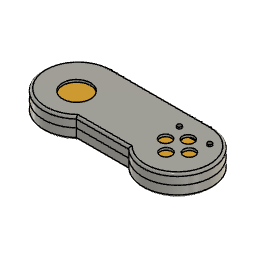
Controller v45 (Autodesk Fusion 360 design; units mm, degrees)
Autodesk Fusion 360 part; units mm, degrees
(part 1 of 2)
sketch "Skizze1" plane through (0, 0, 0) normal (0, 0, 1) x (1, 0, 0)
  line L0 (-75, 23.3) -> (75, 23.3)
  line L1 (75, 23.3) -> (75, -23.3)
  line L2 (75, -23.3) -> (-75, -23.3)
  line L3 (-75, -23.3) -> (-75, 23.3)
  line L4 (-71.7, -23.3) -> (-71.7, -14) construction
  line L5 (-75, -20) -> (-63, -20) construction
  circle A0 centre (-70.1, -18.4) radius 1.6
  line L6 (0, 1.75) -> (0, 22.5) construction
  circle A1 centre (70.1, -18.4) radius 1.6
  line L7 (0, 23.3) -> (0, 21.05) construction
  line L8 (0, 21.05) -> (0, 19.45) construction
  circle A2 centre (0, 19.45) radius 1.6
  line L9 (66.75, 19.8) -> (72.65, 19.8) construction
  line L10 (72.65, 19.8) -> (72.65, 13.9) construction
  line L11 (72.65, 13.9) -> (66.75, 13.9) construction
  line L12 (66.75, 13.9) -> (66.75, 19.8) construction
  line L13 (69.7, 19.8) -> (69.7, 13.9) construction
  circle A3 centre (69.7, 16.85) radius 2.5
  line L14 (34.15, 19.8) -> (40.05, 19.8) construction
  line L15 (40.05, 19.8) -> (40.05, 13.9) construction
  line L16 (40.05, 13.9) -> (34.15, 13.9) construction
  line L17 (34.15, 13.9) -> (34.15, 19.8) construction
  line L18 (37.1, 19.8) -> (37.1, 13.9) construction
  circle A4 centre (37.1, 16.85) radius 2.5
  line L19 (47.25, 16.2) -> (59.15, 16.2) construction
  line L20 (59.15, 16.2) -> (59.15, 4.3) construction
  line L21 (59.15, 4.3) -> (47.25, 4.3) construction
  line L22 (47.25, 4.3) -> (47.25, 16.2) construction
  line L23 (47.25, -7.6) -> (59.15, -7.6) construction
  line L24 (59.15, -7.6) -> (59.15, -19.5) construction
  line L25 (59.15, -19.5) -> (47.25, -19.5) construction
  line L26 (47.25, -19.5) -> (47.25, -7.6) construction
  line L27 (60.1, 4.6) -> (72, 4.6) construction
  line L28 (72, 4.6) -> (72, -7.3) construction
  line L29 (72, -7.3) -> (60.1, -7.3) construction
  line L30 (60.1, -7.3) -> (60.1, 4.6) construction
  line L31 (34.5, 4.6) -> (46.4, 4.6) construction
  line L32 (46.4, 4.6) -> (46.4, -7.3) construction
  line L33 (46.4, -7.3) -> (34.5, -7.3) construction
  line L34 (34.5, -7.3) -> (34.5, 4.6) construction
  line L35 (53.2, 16.2) -> (53.2, 4.3) construction
  line L36 (40.45, 4.6) -> (40.45, -7.3) construction
  line L37 (66.05, 4.6) -> (66.05, -7.3) construction
  line L38 (53.2, -7.6) -> (53.2, -19.5) construction
  circle A5 centre (40.45, -1.35) radius 6.25
  circle A6 centre (53.2, 10.25) radius 6.25
  circle A7 centre (66.05, -1.35) radius 6.25
  circle A8 centre (53.2, -13.55) radius 6.25
  line L39 (-59.6, 3.4) -> (-43.6, 3.4) construction
  line L40 (-43.6, 3.4) -> (-43.6, -12.6) construction
  line L41 (-43.6, -12.6) -> (-59.6, -12.6) construction
  line L42 (-59.6, -12.6) -> (-59.6, 3.4) construction
  line L43 (-51.6, 3.4) -> (-51.6, -12.6) construction
  circle A9 centre (-51.6, -4.6) radius 15
  dimension "d9" = 75
  dimension "d10" = 23.3
  dimension "d11" = 150
  dimension "d12" = 46.6
  dimension "d14" = 3.3
  dimension "d15" = 3.3
  dimension "d16" = 3.2
  dimension "d17" = 2.25
  dimension "d19" = 1.6
  dimension "d20" = 3.2
  dimension "d21" = 5.9
  dimension "d22" = 5.9
  dimension "d23" = 3.5
  dimension "d24" = 2.35
  dimension "d25" = 5
  dimension "d26" = 5.9
  dimension "d27" = 5.9
  dimension "d28" = 3.5
  dimension "d29" = 26.7
  dimension "d30" = 5
  dimension "d33" = 11.9
  dimension "d34" = 11.9
  dimension "d35" = 7.6
  dimension "d36" = 7.1
  dimension "d37" = 11.9
  dimension "d38" = 11.9
  dimension "d39" = 11.9
  dimension "d40" = 11.9
  dimension "d41" = 11.9
  dimension "d42" = 11.9
  dimension "d43" = 11.9
  dimension "d44" = 3
  dimension "d45" = 13.7
  dimension "d46" = 9.3
  dimension "d47" = 12.5
  dimension "d48" = 12.5
  dimension "d49" = 12.5
  dimension "d50" = 12.5
  dimension "d51" = 16
  dimension "d52" = 16
  dimension "d53" = 15.4
  dimension "d54" = 10.7
  dimension "d56" = 30
  constraint horizontal L0
  constraint vertical L1
  constraint horizontal L2
  constraint vertical L3
  constraint coincident L2 L4.start
  constraint perpendicular L2 L4
  constraint coincident L3 L5.start
  constraint perpendicular L3 L5
  constraint tangent L5 A0
  constraint tangent L4 A0
  constraint symmetric A0 L6 A1
  constraint midpoint L0 L7.start
  constraint perpendicular L0 L7
  constraint parallel L6 L8
  constraint coincident L8.end A2.centre
  constraint horizontal L9
  constraint vertical L10
  constraint horizontal L11
  constraint vertical L12
  constraint midpoint L9 L13.start
  constraint midpoint L11 L13.end
  constraint midpoint L13 A3.centre
  constraint horizontal L14
  constraint vertical L15
  constraint horizontal L16
  constraint vertical L17
  constraint midpoint L14 L18.start
  constraint midpoint L16 L18.end
  constraint midpoint L18 A4.centre
  constraint horizontal L19
  constraint vertical L20
  constraint horizontal L21
  constraint vertical L22
  constraint horizontal L23
  constraint vertical L24
  constraint horizontal L25
  constraint vertical L26
  constraint horizontal L27
  constraint vertical L28
  constraint horizontal L29
  constraint vertical L30
  constraint horizontal L31
  constraint vertical L32
  constraint horizontal L33
  constraint vertical L34
  constraint collinear L22 L26
  constraint collinear L27 L31
  constraint midpoint L19 L35.start
  constraint midpoint L21 L35.end
  constraint midpoint L31 L36.start
  constraint midpoint L33 L36.end
  constraint midpoint L27 L37.start
  constraint midpoint L29 L37.end
  constraint midpoint L23 L38.start
  constraint midpoint L25 L38.end
  constraint midpoint L36 A5.centre
  constraint midpoint L35 A6.centre
  constraint midpoint L37 A7.centre
  constraint midpoint L38 A8.centre
  constraint horizontal L39
  constraint vertical L40
  constraint horizontal L41
  constraint vertical L42
  constraint midpoint L39 L43.start
  constraint midpoint L41 L43.end
  constraint midpoint L43 A9.centre
  measures "d9" distance of origin L3
  measures "d10" distance of origin L0
  measures "d11" distance of L0.start L0.end
  measures "d12" distance of L0.start L2.end
  measures "d14" distance of L3 L4
  measures "d15" distance of L2 L5
  measures "d16" diameter of A0
  measures "d17" distance of L7.start L7.end
  measures "d19" distance of L7.end L8.end
  measures "d20" diameter of A2
  measures "d21" distance of L9.start L9.end
  measures "d22" distance of L9.start L11.end
  measures "d23" distance of L0 L9
  measures "d24" distance of L1 L10
  measures "d25" diameter of A3
  measures "d26" distance of L14.start L14.end
  measures "d27" distance of L14.start L16.end
  measures "d28" distance of L0 L14
  measures "d29" distance of L12 L15
  measures "d30" diameter of A4
  measures "d33" distance of L19.start L19.end
  measures "d34" distance of L19.start L21.end
  measures "d35" distance of L12 L20
  measures "d36" distance of L0 L19
  measures "d37" distance of L23.start L23.end
  measures "d38" distance of L23.start L25.end
  measures "d39" distance of L27.start L27.end
  measures "d40" distance of L27.start L29.end
  measures "d41" distance of L31.start L31.end
  measures "d42" distance of L31.start L33.end
  measures "d43" distance of L21 L23
  measures "d44" distance of L1 L28
  measures "d45" distance of L30 L32
  measures "d46" distance of L11 L27
  measures "d47" diameter of A5
  measures "d48" diameter of A6
  measures "d49" diameter of A7
  measures "d50" diameter of A8
  measures "d51" distance of L39.start L39.end
  measures "d52" distance of L39.start L41.end
  measures "d53" distance of L3 L42
  measures "d54" distance of L2 L41
  measures "d56" diameter of A9
sketch "Skizze2" plane through (0, 0, 0) normal (0, 0, 1) x (1, 0, 0)
  circle A0 centre (-51.6, -4.6) radius 15
  circle A1 centre (40.45, -1.35) radius 6.25
  circle A2 centre (53.2, 10.25) radius 6.25
  circle A3 centre (66.05, -1.35) radius 6.25
  circle A4 centre (53.2, -13.55) radius 6.25
  circle A5 centre (69.7, 16.85) radius 2.5
  circle A6 centre (37.1, 16.85) radius 2.5
  circle A7 centre (70.1, -18.4) radius 1.6
  circle A8 centre (0, 19.45) radius 1.6
  circle A9 centre (-70.1, -18.4) radius 1.6
  line L0 (-75, -23.3) -> (-75, 23.3)
  line L1 (-75, 23.3) -> (75, 23.3)
  line L2 (75, 23.3) -> (75, -23.3)
  line L3 (75, -23.3) -> (-75, -23.3)
  line L4 (40.45, -1.35) -> (66.05, -1.35) construction
  line L5 (53.2, 10.25) -> (53.2, -13.55) construction
  circle A10 centre (53.25, -1.35) radius 32.8738 construction
  line L6 (0, 87.6668) -> (0, -41.0668) construction
  circle A11 centre (53.25, -1.35) radius 36.8738 construction
  line L7 (53.25, 35.5238) -> (0, 35.5238)
  line L8 (28.0831, -28.3) -> (0, -28.3)
  arc A12 (28.0831, -28.3) -> (53.25, 35.5238) centre (53.25, -1.35) ccw
  line L9 (-53.25, 35.5238) -> (0, 35.5238)
  arc A13 (-53.25, 35.5238) -> (-28.0831, -28.3) centre (-53.25, -1.35) ccw
  line L10 (-28.0831, -28.3) -> (0, -28.3)
  dimension "d59" = 4
  dimension "d60" = 5
  constraint coincident A1.centre L4.start
  constraint coincident A3.centre L4.end
  constraint coincident A2.centre L5.start
  constraint coincident A4.centre L5.end
  constraint midpoint L4 A10.centre
  constraint coincident L1.end A10
  constraint perpendicular L3 L6
  constraint midpoint L1 L6
  constraint coincident A11 L7.start
  constraint coincident L6 L7.end
  constraint tangent A11 L7
  constraint coincident A11 L8.start
  constraint coincident L6 L8.end
  constraint perpendicular L6 L8
  constraint perpendicular L6 L7
  constraint tangent L7 A12
  constraint symmetric L6 L7.start L9.start
  constraint symmetric L6 L7.end L9.end
  constraint symmetric L6 L8.start A13.end
  constraint symmetric L6 L8.end L10.end
  constraint symmetric L6 A12 A13
  measures "d60" distance of L3 L8
sketch "Skizze3" plane through (0, 0, 0) normal (0, 0, 1) x (1, 0, 0)
  line L0 (-53.25, 35.5238) -> (0, 35.5238)
  arc A0 (-53.25, 35.5238) -> (-28.0831, -28.3) centre (-53.25, -1.35) ccw
  line L1 (-28.0831, -28.3) -> (0, -28.3)
  line L2 (28.0831, -28.3) -> (0, -28.3)
  arc A1 (28.0831, -28.3) -> (53.25, 35.5238) centre (53.25, -1.35) ccw
  line L3 (53.25, 35.5238) -> (0, 35.5238)
  line L4 (-75, 23.3) -> (75, 23.3) construction
  line L5 (-75, -23.3) -> (-75, 23.3) construction
  line L6 (75, -23.3) -> (-75, -23.3) construction
  line L7 (75, 23.3) -> (75, -23.3) construction
  arc A2 (-53.25, 33.0238) -> (-29.089, -25.8) centre (-53.25, -1.35) ccw
  line L8 (-29.089, -25.8) -> (0, -25.8)
  line L9 (29.089, -25.8) -> (0, -25.8)
  arc A3 (29.089, -25.8) -> (53.25, 33.0238) centre (53.25, -1.35) ccw
  line L10 (53.25, 33.0238) -> (0, 33.0238)
  line L11 (-53.25, 33.0238) -> (0, 33.0238)
  circle A4 centre (-70.1, -18.4) radius 1.25
  circle A5 centre (-70.1, -18.4) radius 3
  circle A6 centre (0, 19.45) radius 1.5
  circle A7 centre (0, 19.45) radius 3
  circle A8 centre (70.1, -18.4) radius 3
  circle A9 centre (70.1, -18.4) radius 1.25
  circle A10 centre (0, 19.45) radius 5.5
  circle A11 centre (-70.1, -18.4) radius 5.5
  circle A12 centre (70.1, -18.4) radius 5.5
  circle A13 centre (83.25, 0) radius 2.75
  circle A14 centre (83.25, 0) radius 1.75
  line L12 (78, 22.5036) -> (78, -25.2036)
  line L13 (0, -28.3) -> (0, 35.5238) construction
  line L14 (-78, 22.5036) -> (-78, -25.2036)
  circle A15 centre (-83.25, 0) radius 2.75
  circle A16 centre (-83.25, 0) radius 1.75
  point P0 (0, 19.45)
  point P1 (70.1, -18.4)
  point P2 (-70.1, -18.4)
  dimension "d62" = 2.5
  dimension "d63" = 6
  dimension "d64" = 3
  dimension "d65" = 6
  dimension "d66" = 6
  dimension "d67" = 2.5
  dimension "d69" = 2.5
  dimension "d70" = 2.5
  dimension "d71" = 2.5
  dimension "d257" = 5.5
  dimension "d258" = 3.5
  dimension "d261" = 3
  dimension "d262" = 5.25
  constraint coincident P2 A4.centre
  constraint coincident P0 A6.centre
  constraint concentric A6 A7
  constraint coincident P1 A8.centre
  constraint concentric A8 A9
  constraint concentric A13 A14
  constraint coincident A3 L12.start
  constraint coincident A3 L12.end
  constraint vertical L12
  constraint coincident L1.end L2.end
  constraint coincident L0.end L3.end
  constraint symmetric A13 L13 A15
  constraint symmetric A14 L13 A16
  constraint symmetric L12.start L13 L14.start
  constraint symmetric L12.end L13 L14.end
  measures "d62" diameter of A4
  measures "d63" diameter of A5
  measures "d64" diameter of A6
  measures "d65" diameter of A7
  measures "d66" diameter of A8
  measures "d67" diameter of A9
  measures "d257" diameter of A13
  measures "d258" diameter of A14
  measures "d261" distance of L7 L12
  measures "d262" distance of A13.centre L12
extrude "Extrusion1" add sketch "Skizze3" along normal blind 2.5 contours A2 L8 L9 A3 L10 L11 L12 L14 | A2 L14 | A3 L12 makes body 1
extrude "Extrusion2" add sketch "Skizze3" along normal blind 10 contours A5 | A7 | A8 | A10 | A11 | A12 bodies 1
extrude "Extrusion3" cut sketch "Skizze3" along normal blind 6.25 contours A5 | A7 | A8 bodies 1
extrude "Extrusion4" add sketch "Skizze3" along normal blind 11.5 separate body contours L0 A0 L1 L2 A1 L3 | A2 L14 | A3 L12 | A13 | A14 | A15 | A16 makes body 2
extrude "Extrusion28" cut sketch "Skizze3" along normal blind 11.5 contours A14 | A16 bodies 2
extrude "Extrusion29" cut sketch "Skizze3" along normal blind 5 contours A13 | A15 bodies 2
sketch "Skizze4" plane through (0, 0, 10) normal (0, 0, 1) x (-1, 0, 0)
  circle A0 centre (0, -19.45) radius 1.5
  circle A1 centre (0, -19.45) radius 5.5
  line L0 (75, -23.3) -> (-75, -23.3)
  line L1 (75, 23.3) -> (75, -23.3)
  line L2 (-75, 23.3) -> (75, 23.3)
  line L3 (-75, -23.3) -> (-75, 23.3)
  circle A2 centre (-37.1, -16.85) radius 2.5
  circle A3 centre (-53.2, -10.25) radius 6.25
  circle A4 centre (-69.7, -16.85) radius 2.5
  circle A5 centre (-66.05, 1.35) radius 6.25
  circle A6 centre (-40.45, 1.35) radius 6.25
  circle A7 centre (-53.2, 13.55) radius 6.25
  circle A8 centre (51.6, 4.6) radius 15
extrude "Extrusion5" add sketch "Skizze4" along normal blind 1.6 separate body contours A1 L0 | A1 L0 L1 L2 L3 | A2 | A3 | A4 | A5 | A6 | A7 | A8 picked at (-0.0374, -22.5153) makes body 3
ref_plane "Arbeitsebene1" through (0, 0, 22.2) normal (0, 0, 1) x (1, 0, 0)
sketch "Skizze7" plane through (0, 0, 22.2) normal (0, 0, 1) x (1, 0, 0)
  circle A0 centre (-51.6, -4.6) radius 15
  circle A1 centre (53.2, -13.55) radius 6.25
  circle A2 centre (40.45, -1.35) radius 6.25
  circle A3 centre (53.2, 10.25) radius 6.25
  circle A4 centre (37.1, 16.85) radius 2.5
  circle A5 centre (66.05, -1.35) radius 6.25
  circle A6 centre (69.7, 16.85) radius 2.5
  circle A7 centre (0, 19.45) radius 1.5
  circle A8 centre (0, 19.45) radius 2.75
  circle A9 centre (-70.1, -18.4) radius 1.5
  circle A10 centre (-70.1, -18.4) radius 4
  circle A11 centre (70.1, -18.4) radius 1.5
  circle A12 centre (70.1, -18.4) radius 4
  line L0 (-53.25, 35.5238) -> (0, 35.5238)
  arc A13 (-53.25, 35.5238) -> (-28.0831, -28.3) centre (-53.25, -1.35) ccw
  arc A14 (-53.25, 33.0238) -> (-29.089, -25.8) centre (-53.25, -1.35) ccw construction
  line L1 (-53.25, 33.0238) -> (0, 33.0238) construction
  line L2 (53.25, 35.5238) -> (0, 35.5238)
  line L3 (53.25, 33.0238) -> (0, 33.0238) construction
  arc A15 (28.0831, -28.3) -> (53.25, 35.5238) centre (53.25, -1.35) ccw
  arc A16 (29.089, -25.8) -> (53.25, 33.0238) centre (53.25, -1.35) ccw construction
  line L4 (29.089, -25.8) -> (0, -25.8)
  line L5 (28.0831, -28.3) -> (0, -28.3)
  line L6 (-28.0831, -28.3) -> (0, -28.3)
  line L7 (-29.089, -25.8) -> (0, -25.8)
  line L8 (-53.25, 33.0238) -> (-53.25, 35.5238)
  line L9 (53.25, 33.0238) -> (53.25, 35.5238)
  line L10 (0, 35.5238) -> (0, 33.0238) construction
  line L11 (-28.25, 35.5238) -> (-28.25, 33.0238)
  line L12 (-28.25, 33.0238) -> (-23.25, 33.0238)
  line L13 (-23.25, 33.0238) -> (-23.25, 30.5238)
  line L14 (-23.25, 30.5238) -> (-30.75, 30.5238)
  line L15 (-30.75, 33.0238) -> (-53.25, 33.0238) construction
  line L16 (-20.75, 33.0238) -> (-20.75, 28.0238)
  line L17 (-20.75, 28.0238) -> (-30.75, 28.0238)
  line L18 (-20.75, 33.0238) -> (0, 33.0238)
  line L19 (53.25, 33.0238) -> (53.25, 35.5238)
  line L20 (30.75, 33.0238) -> (53.25, 33.0238) construction
  line L21 (28.25, 35.5238) -> (28.25, 33.0238)
  line L22 (28.25, 33.0238) -> (23.25, 33.0238)
  line L23 (23.25, 33.0238) -> (23.25, 30.5238)
  line L24 (20.75, 33.0238) -> (20.75, 28.0238)
  line L25 (20.75, 33.0238) -> (0, 33.0238)
  line L26 (20.75, 28.0238) -> (30.75, 28.0238)
  line L27 (23.25, 30.5238) -> (30.75, 30.5238)
  line L28 (-50.25, 33.0238) -> (-44.25, 33.0238) construction
  line L29 (-44.25, 33.0238) -> (-44.25, 28.0238) construction
  line L30 (-44.25, 28.0238) -> (-50.25, 28.0238) construction
  line L31 (-50.25, 28.0238) -> (-50.25, 33.0238) construction
  line L32 (-53.25, 31.3238) -> (-50.25, 31.3238)
  line L33 (-50.25, 31.3238) -> (-50.25, 29.8238)
  line L34 (-50.25, 29.8238) -> (-52.824, 29.8238)
  line L35 (-53.25, 31.3238) -> (-53.25, 33.0238)
  line L36 (-52.824, 29.8238) -> (-67.7328, 29.8238)
  line L37 (-47.25, 33.0238) -> (-47.25, 28.0238) construction
  line L38 (-41.25, 31.3238) -> (-44.25, 31.3238)
  line L39 (-44.25, 31.3238) -> (-44.25, 29.8238)
  line L40 (-44.25, 29.8238) -> (-41.676, 29.8238)
  line L41 (-41.25, 31.3238) -> (-30.75, 30.5238)
  line L42 (-41.676, 29.8238) -> (-30.75, 28.0238)
  line L43 (-47.25, 28.0238) -> (-49.75, 28.0238)
  line L44 (-47.25, 28.0238) -> (-44.75, 28.0238)
  line L45 (-75, 23.3) -> (75, 23.3) construction
  line L46 (-49.75, 28.0238) -> (-49.75, 24.0238)
  line L47 (-49.75, 24.0238) -> (-44.75, 24.0238)
  line L48 (-44.75, 24.0238) -> (-44.75, 28.0238)
  arc A17 (-67.7328, 29.8238) -> (-29.089, -25.8) centre (-53.25, -1.35) ccw
  line L49 (41.676, 29.8238) -> (30.75, 28.0238)
  line L50 (41.25, 31.3238) -> (30.75, 30.5238)
  line L51 (41.25, 31.3238) -> (44.25, 31.3238)
  line L52 (44.25, 31.3238) -> (44.25, 29.8238)
  line L53 (44.25, 29.8238) -> (41.676, 29.8238)
  line L54 (47.25, 28.0238) -> (44.75, 28.0238)
  line L55 (47.25, 28.0238) -> (49.75, 28.0238)
  line L56 (49.75, 28.0238) -> (49.75, 24.0238)
  line L57 (49.75, 24.0238) -> (44.75, 24.0238)
  line L58 (44.75, 24.0238) -> (44.75, 28.0238)
  line L59 (53.25, 31.3238) -> (53.25, 33.0238)
  line L60 (53.25, 31.3238) -> (50.25, 31.3238)
  line L61 (50.25, 31.3238) -> (50.25, 29.8238)
  line L62 (50.25, 29.8238) -> (52.824, 29.8238)
  line L63 (52.824, 29.8238) -> (67.7328, 29.8238)
  arc A18 (29.089, -25.8) -> (67.7328, 29.8238) centre (53.25, -1.35) ccw
  line L64 (2.75, 33.0238) -> (2.75, -0.1762) construction
  line L65 (2.75, -0.1762) -> (20.75, -0.1762) construction
  line L66 (20.75, -0.1762) -> (20.75, 28.0238) construction
  line L67 (7.5, 33.0238) -> (7.5, 35.5238)
  line L68 (16, 33.0238) -> (16, 35.5238)
  line L69 (2.75, 33.0238) -> (20.75, 33.0238) construction
  line L70 (7.5, 34.2738) -> (16, 34.2738) construction
  line L71 (11.75, 34.2738) -> (11.75, 33.0238) construction
  circle A19 centre (-83.25, 0) radius 2.75
  circle A20 centre (-83.25, 0) radius 1.75
  line L72 (-78, 22.5036) -> (-78, -25.2036)
  circle A21 centre (83.25, 0) radius 2.75
  circle A22 centre (83.25, 0) radius 1.75
  line L73 (78, 22.5036) -> (78, -25.2036)
  circle A23 centre (-83.25, 0) radius 1.45
  circle A24 centre (83.25, 0) radius 1.45
  line L74 (16.75, 33.0238) -> (16.75, -0.1762)
  line L75 (6.75, 33.0238) -> (6.75, -0.1762)
  line L76 (16.75, -0.1762) -> (6.75, -0.1762)
  line L77 (16.75, -0.1762) -> (16.75, -5.1762)
  line L78 (16.75, -5.1762) -> (6.75, -5.1762)
  line L79 (6.75, -5.1762) -> (6.75, -0.1762)
  point P0 (-70.1, -18.4)
  point P1 (0, 19.45)
  point P2 (70.1, -18.4)
  dimension "d107" = 3
  dimension "d109" = 3
  dimension "d110" = 8
  dimension "d111" = 3
  dimension "d112" = 8
  dimension "d122" = 25
  dimension "d125" = 5
  dimension "d126" = 2.5
  dimension "d127" = 7.5
  dimension "d128" = 2.5
  dimension "d134" = 6
  dimension "d135" = 5
  dimension "d136" = 1.7
  dimension "d138" = 1.5
  dimension "d139" = 3
  dimension "d140" = 2.5
  dimension "d141" = 2.5
  dimension "d142" = 4
  dimension "d148" = 33.2
  dimension "d149" = 18
  dimension "d150" = 6.5
  dimension "d174" = 8.5
  dimension "d269" = -0.3
  dimension "d270" = -0.3
  dimension "d273" = 10
  dimension "d274" = 5
  dimension "d275" = 5
  constraint coincident P1 A7.centre
  constraint concentric A7 A8
  constraint coincident P0 A9.centre
  constraint coincident P2 A11.centre
  constraint concentric A11 A12
  constraint coincident A14.start L1.start
  constraint coincident L0.start A13.start
  constraint coincident L3.start A16.end
  constraint coincident L2.start A15.end
  constraint coincident L0.end L2.end
  constraint coincident L1.end L3.end
  constraint coincident L0 L11.start
  constraint coincident L1 L11.end
  constraint perpendicular L1 L11
  constraint perpendicular L11 L12
  constraint perpendicular L1 L13
  constraint perpendicular L11 L14
  constraint perpendicular L10 L18
  constraint symmetric A14.start L10 L3.start
  constraint symmetric L0.start L10 L2.start
  constraint symmetric L1.end L10 L3.end
  constraint symmetric L10 L11.start L21.start
  constraint symmetric L10 L11.end L21.end
  constraint symmetric L10 L12.end L22.end
  constraint symmetric L10 L13.end L23.end
  constraint symmetric L10 L14.end L27.end
  constraint symmetric L10 L15.start L20.start
  constraint symmetric L10 A14.start L3.start
  constraint symmetric L10 L16.start L24.start
  constraint symmetric L10 L16.end L24.end
  constraint symmetric L10 L17.end L26.end
  constraint horizontal L28
  constraint vertical L29
  constraint horizontal L30
  constraint vertical L31
  constraint collinear L15 L28
  constraint horizontal L32
  constraint vertical L33
  constraint horizontal L34
  constraint collinear L31 L33
  constraint coincident A14 L36.end
  constraint midpoint L28 L37.start
  constraint midpoint L30 L37.end
  constraint symmetric L32.start L37 L38.start
  constraint symmetric L32.end L37 L38.end
  constraint symmetric L33.end L37 L39.end
  constraint symmetric L34.end L37 L40.end
  constraint perpendicular L37 L43
  constraint perpendicular L37 L44
  constraint perpendicular L43 L46
  constraint perpendicular L46 L47
  constraint perpendicular L30 L48
  constraint coincident A14.end L7.start
  constraint coincident A13.centre A14.centre
  constraint symmetric L10 L32.start L59.start
  constraint symmetric L10 L32.end L60.end
  constraint symmetric L10 L33.end L61.end
  constraint symmetric L10 L34.end L62.end
  constraint symmetric L10 L36.end L63.end
  constraint symmetric L10 L37.end L54.start
  constraint symmetric L10 L38.start L50.start
  constraint symmetric L10 L38.end L51.end
  constraint symmetric L10 L39.end L52.end
  constraint symmetric L10 L40.end L49.start
  constraint symmetric L10 L43.end L55.end
  constraint symmetric L10 L44.end L54.end
  constraint symmetric L10 L46.end L56.end
  constraint symmetric L10 L47.end L57.end
  constraint symmetric L10 A14.end A16.start
  constraint symmetric L10 A17 A18
  constraint coincident L3 L64.start
  constraint perpendicular L45 L64
  constraint tangent A8 L64
  constraint perpendicular L24 L65
  constraint perpendicular L26 L66
  constraint coincident L25 L67.start
  constraint coincident L2 L67.end
  constraint perpendicular L2 L67
  constraint coincident L3 L68.start
  constraint coincident L2 L68.end
  constraint perpendicular L2 L68
  constraint midpoint L67 L70.start
  constraint midpoint L68 L70.end
  constraint midpoint L70 L71.start
  constraint midpoint L69 L71.end
  constraint perpendicular L69 L71
  constraint coincident L3 L74.start
  constraint coincident L65 L74.end
  constraint perpendicular L65 L74
  constraint coincident L25 L75.start
  constraint coincident L65 L75.end
  constraint perpendicular L65 L75
  constraint perpendicular L76 L77
  constraint perpendicular L75 L78
  constraint perpendicular L76 L79
  measures "d107" diameter of A7
  measures "d109" diameter of A9
  measures "d110" diameter of A10
  measures "d111" diameter of A11
  measures "d112" diameter of A12
  measures "d122" distance of L8 L11
  measures "d125" distance of L11.end L12.end
  measures "d126" distance of L12.end L13.end
  measures "d127" distance of L13.end L14.end
  measures "d128" distance of L14.end L15.start
  measures "d134" distance of L28.start L28.end
  measures "d135" distance of L28.start L30.end
  measures "d136" distance of L15 L32
  measures "d138" distance of L32 L34
  measures "d139" distance of L33 L35
  measures "d140" distance of L37.end L43.end
  measures "d141" distance of L37.end L44.end
  measures "d142" distance of L43.end L46.end
  measures "d148" distance of L64.start L64.end
  measures "d149" distance of L24 L64
  measures "d174" distance of L67 L68
  measures "d273" distance of L74 L75
  measures "d274" distance of L71 L74
  measures "d275" distance of L74.end L77.end
extrude "Extrusion7" add sketch "Skizze7" against normal blind 2.5 separate body contours A7 | A9 | A11 | L0 L2 L4 L7 L8 L9 L11 L12 L13 L14 L16 L17 L18 L19 L21 L22 L23 L24 L25 L26 L27 L32 L33 L34 L35 L36 L38 L39 L40 L41 L42 A17 L49 L50 L51 L52 L53 L59 L60 L61 L62 L63 A18 L72 L73 L74 L75 L77 L78 L79 | L25 L74 L75 L76 | L76 L77 L78 L79 | L43 L44 L46 L47 L48 | L54 L55 L56 L57 L58 makes body 4 at (-69.1075, -17.2753, 20.5333) makes body 5 at (1.4981, 19.3752, 20.5333) makes body 6 at (0.0685, -11.6308, 22.2) makes body 7 at (71.0925, -17.2753, 20.5333)
extrude "Extrusion8" add sketch "Skizze7" against normal blind 10.6 contours A8 | A10 | A12 bodies 4 5 6 7
extrude "Extrusion12" add sketch "Skizze7" against normal blind 10.7 separate body contours A13 A15 L4 L5 L6 L7 L8 L9 L19 L32 L33 L34 L35 L36 A17 L59 L60 L61 L62 L63 A18 | L0 L2 L11 L12 L13 L14 L16 L17 L18 L25 L38 L39 L40 L41 L42 L67 | L2 L25 L67 L68 | L2 L21 L22 L23 L24 L25 L26 L27 L49 L50 L51 L52 L53 L68 | A17 L72 | A18 L73 | L43 L44 L46 L47 L48 | L54 L55 L56 L57 L58 | A19 | A20 | A21 | A22 makes body 8 at (-48.0833, 28.0238, 18.6333) makes body 9 at (9.4167, 35.5238, 15.0667) makes body 10 at (55.0895, 35.4779, 15.0667) makes body 11 at (46.4167, 28.0238, 18.6333)
extrude "Extrusion30" add sketch "Skizze7" against normal blind 2.5 separate body contours A23 | A24 makes body 12 at (-84.5234, 0.6935, 20.5333) makes body 13 at (81.9766, 0.6935, 20.5333)
sketch "Skizze8" plane through (0, 35.5238, 0) normal (0, 1, 0) x (-1, 0, 0)
  line L0 (28.25, 22.2) -> (-28.25, 22.2)
  line L1 (-28.25, 22.2) -> (-28.25, 11.5)
  line L2 (-28.25, 11.5) -> (28.25, 11.5)
  line L3 (28.25, 11.5) -> (28.25, 22.2)
  line L4 (-16, 14.5) -> (-7.5, 14.5)
  line L5 (-7.5, 14.5) -> (-7.5, 11.5)
  line L6 (-7.5, 11.5) -> (-16, 11.5)
  line L7 (-16, 11.5) -> (-16, 14.5)
  line L8 (-16, 22.2) -> (-16, 14.5) construction
  line L9 (-7.5, 22.2) -> (-7.5, 14.5) construction
  line L10 (-7.5, 22.2) -> (-16, 22.2)
  line L11 (6.65, 14.2) -> (16.85, 14.2)
  line L12 (16.85, 14.2) -> (16.85, 11.5)
  line L13 (16.85, 11.5) -> (6.65, 11.5)
  line L14 (6.65, 11.5) -> (6.65, 14.2)
  line L15 (-11.75, 14.5) -> (-11.75, 11.5) construction
  line L16 (0, 22.2) -> (0, 11.5)
  line L17 (11.75, 14.5) -> (11.75, 11.5) construction
  line L18 (-19, 17.5) -> (-4.5, 17.5)
  line L19 (-4.5, 17.5) -> (-4.5, 8.5)
  line L20 (-4.5, 8.5) -> (-19, 8.5)
  line L21 (-19, 8.5) -> (-19, 17.5)
  line L22 (6.65, 14.2) -> (6.65, 18.2) construction
  line L23 (9.2, 14.2) -> (9.2, 18.2) construction
  line L24 (11.75, 14.2) -> (11.75, 18.2) construction
  line L25 (14.3, 14.2) -> (14.3, 18.2) construction
  line L26 (16.85, 14.2) -> (16.85, 18.2) construction
  line L27 (18.35, 14.2) -> (18.35, 11.5)
  line L28 (5.15, 11.5) -> (5.15, 14.2)
  line L29 (20.75, 19.7) -> (-20.75, 19.7)
  line L30 (5.15, 14.2) -> (5.15, 19.7)
  line L31 (18.35, 14.2) -> (18.35, 19.7)
  line L32 (5.15, 11.5) -> (6.65, 11.5)
  line L33 (16.85, 11.5) -> (18.35, 11.5)
  circle A0 centre (11.75, 5.9217) radius 2.8
  line L34 (11.75, 11.5) -> (11.75, 0.3434) construction
  circle A1 centre (11.75, 5.9217) radius 4.8 construction
  line L35 (6.95, 0) -> (6.95, 5.9217)
  line L36 (16.55, 0) -> (16.55, 5.9217)
  arc A2 (16.55, 5.9217) -> (6.95, 5.9217) centre (11.75, 5.9217) ccw
  line L37 (6.95, 0) -> (16.55, 0)
  point P0 (-16, 22.2)
  point P1 (-7.5, 22.2)
  point P2 (0, 22.2)
  dimension "d179" = 3
  dimension "d182" = 2.7
  dimension "d183" = 10.2
  dimension "d184" = 5.1
  dimension "d188" = 3
  dimension "d190" = 3
  dimension "d191" = 3
  dimension "d192" = 3
  dimension "d202" = 4
  dimension "d205" = 10.2
  dimension "d206" = 0
  dimension "d218" = -1.5
  dimension "d219" = -1.5
  dimension "d240" = 5.6
  dimension "d241" = 2
  dimension "d281" = 4.7
  constraint horizontal L4
  constraint vertical L5
  constraint horizontal L6
  constraint vertical L7
  constraint collinear L2 L6
  constraint coincident P0 L8.start
  constraint coincident P1 L9.start
  constraint perpendicular L9 L10
  constraint perpendicular L8 L10
  constraint horizontal L11
  constraint vertical L12
  constraint horizontal L13
  constraint vertical L14
  constraint midpoint L4 L15.start
  constraint midpoint L6 L15.end
  constraint coincident P2 L16.start
  constraint midpoint L2 L16.end
  constraint symmetric L15.start L16 L17.start
  constraint symmetric L15.end L16 L17.end
  constraint collinear L2 L13
  constraint horizontal L18
  constraint vertical L19
  constraint horizontal L20
  constraint vertical L21
  constraint perpendicular L11 L22
  constraint coincident L29 L30.end
  constraint perpendicular L29 L30
  constraint coincident L29 L31.end
  constraint perpendicular L29 L31
  constraint perpendicular L14 L32
  constraint perpendicular L13 L34
  constraint midpoint A0.centre L34
  constraint coincident A1 L35.end
  constraint coincident A1 L36.end
  constraint vertical L35
  constraint vertical L36
  constraint tangent A1 L35
  constraint tangent A1 L36
  constraint coincident A0.centre A1.centre
  constraint perpendicular L36 L37
  measures "d179" distance of L4 L6
  measures "d182" distance of L11 L13
  measures "d183" distance of L12 L14
  measures "d184" distance of L14 L17
  measures "d188" distance of L4 L18
  measures "d190" distance of L7 L21
  measures "d191" distance of L5 L19
  measures "d192" distance of L6 L20
  measures "d202" distance of L11.start L22.end
  measures "d240" diameter of A0
  measures "d281" distance of L0 L18
sketch "Skizze9" plane through (0, 0, 19.7) normal (0, 0, -1) x (1, 0, 0)
  line L0 (-53.25, -35.5238) -> (-28.25, -35.5238) construction
  circle A0 centre (-51.6, 4.6) radius 15 construction
  circle A1 centre (53.2, 13.55) radius 6.25 construction
  circle A2 centre (40.45, 1.35) radius 6.25 construction
  circle A3 centre (53.2, -10.25) radius 6.25 construction
  circle A4 centre (37.1, -16.85) radius 2.5 construction
  circle A5 centre (66.05, 1.35) radius 6.25 construction
  circle A6 centre (69.7, -16.85) radius 2.5 construction
  circle A7 centre (0, -19.45) radius 2.75 construction
  circle A8 centre (-70.1, 18.4) radius 4 construction
  circle A9 centre (70.1, 18.4) radius 4 construction
  line L1 (53.25, -31.3238) -> (53.25, -35.5238) construction
  line L2 (50.25, -31.3238) -> (53.25, -31.3238) construction
  line L3 (41.25, -31.3238) -> (44.25, -31.3238) construction
  line L4 (30.75, -30.5238) -> (41.25, -31.3238) construction
  line L5 (23.25, -30.5238) -> (30.75, -30.5238) construction
  line L6 (23.25, -33.0238) -> (23.25, -30.5238) construction
  line L7 (28.25, -35.5238) -> (28.25, -33.0238) construction
  line L8 (28.25, -33.0238) -> (23.25, -33.0238) construction
  line L9 (-28.25, -35.5238) -> (28.25, -35.5238) construction
  arc A10 (53.25, -35.5238) -> (28.0831, 28.3) centre (53.25, 1.35) ccw construction
  line L10 (52.75, -36.0238) -> (28.75, -36.0238)
  line L11 (28.75, -36.0238) -> (28.75, -32.7738)
  line L12 (28.75, -32.7738) -> (23.5, -32.7738)
  line L13 (23.5, -32.7738) -> (23.5, -30.7738)
  line L14 (23.5, -30.7738) -> (31.25, -30.7738)
  line L15 (31.25, -30.7738) -> (31.25, -34.5238)
  line L16 (52.75, -34.5238) -> (52.75, -36.0238)
  line L17 (47.25, -28.0238) -> (44.75, -28.0238) construction
  line L18 (47.25, -28.0238) -> (49.75, -28.0238) construction
  line L19 (47.25, -33.0238) -> (49.75, -33.0238)
  line L20 (47.25, -33.0238) -> (44.75, -33.0238)
  line L21 (52.75, -34.5238) -> (49.75, -34.5238)
  line L22 (49.75, -33.0238) -> (49.75, -34.5238)
  line L23 (44.75, -33.0238) -> (44.75, -34.5238)
  line L24 (44.75, -34.5238) -> (31.25, -34.5238)
  line L25 (0, -35.5238) -> (0, -33.0238) construction
  line L26 (-28.25, -35.0238) -> (-53.25, -35.0238) construction
  line L27 (-44.25, -29.8238) -> (-44.25, -31.3238) construction
  line L28 (-23.25, -30.5238) -> (-30.75, -30.5238) construction
  line L29 (-28.25, -35.5238) -> (-28.25, -33.0238) construction
  line L30 (-30.75, -30.5238) -> (-41.25, -31.3238) construction
  line L31 (-28.25, -33.0238) -> (-23.25, -33.0238) construction
  line L32 (-44.75, -34.5238) -> (-31.25, -34.5238)
  line L33 (-28.75, -36.0238) -> (-28.75, -32.7738)
  line L34 (-23.5, -32.7738) -> (-23.5, -30.7738)
  line L35 (-52.75, -34.5238) -> (-52.75, -36.0238)
  line L36 (-23.5, -30.7738) -> (-31.25, -30.7738)
  line L37 (-52.75, -34.5238) -> (-49.75, -34.5238)
  line L38 (-47.25, -28.0238) -> (-49.75, -28.0238) construction
  line L39 (-44.25, -31.3238) -> (-41.25, -31.3238) construction
  line L40 (-31.25, -30.7738) -> (-31.25, -34.5238)
  line L41 (-28.75, -32.7738) -> (-23.5, -32.7738)
  line L42 (-23.25, -31.0238) -> (-23.25, -33.0238) construction
  line L43 (-21.25, -29.0238) -> (-30.25, -29.0238) construction
  line L44 (-30.25, -31.0238) -> (-23.25, -31.0238) construction
  line L45 (-21.25, -33.0238) -> (-21.25, -29.0238) construction
  line L46 (-41.25, -31.3238) -> (-30.25, -31.0238) construction
  line L47 (-30.25, -29.0238) -> (-41.25, -29.8238) construction
  line L48 (-47.25, -28.0238) -> (-44.75, -28.0238) construction
  line L49 (-47.25, -33.0238) -> (-44.75, -33.0238)
  line L50 (-49.75, -33.0238) -> (-49.75, -34.5238)
  line L51 (-50.25, -31.3238) -> (-53.25, -31.3238) construction
  line L52 (-23.25, -33.0238) -> (-23.25, -30.5238) construction
  line L53 (-47.25, -33.0238) -> (-49.75, -33.0238)
  line L54 (-41.25, -31.3238) -> (-44.25, -31.3238) construction
  line L55 (-53.25, -35.0238) -> (-53.25, -31.3238) construction
  line L56 (-41.25, -29.8238) -> (-44.25, -29.8238) construction
  line L57 (-52.75, -36.0238) -> (-28.75, -36.0238)
  line L58 (-23.25, -33.0238) -> (-28.25, -33.0238) construction
  line L59 (-44.75, -33.0238) -> (-44.75, -34.5238)
  line L60 (-53.25, -31.3238) -> (-50.25, -31.3238) construction
  line L61 (-28.25, -33.0238) -> (-28.25, -35.0238) construction
  line L62 (-50.25, -31.3238) -> (-50.25, -29.8238) construction
  line L63 (-53.25, -31.3238) -> (-53.25, -35.5238) construction
  line L64 (44.25, -31.9238) -> (41.25, -31.9238) construction
  line L65 (-50.25, -31.3238) -> (-53.25, -31.3238)
  line L66 (-53.25, -31.3238) -> (-53.25, -35.5238)
  line L67 (-28.25, -35.5238) -> (-28.25, -33.0238)
  line L68 (-28.25, -33.0238) -> (-23.25, -33.0238)
  line L69 (-23.25, -33.0238) -> (-23.25, -30.5238)
  line L70 (-23.25, -30.5238) -> (-30.75, -30.5238)
  line L71 (-30.75, -30.5238) -> (-41.25, -31.3238)
  line L72 (-41.25, -31.3238) -> (-44.25, -31.3238)
  line L73 (-44.25, -31.3238) -> (-44.25, -29.8238)
  line L74 (-44.25, -29.8238) -> (-41.676, -29.8238)
  line L75 (-41.676, -29.8238) -> (-30.75, -28.0238)
  line L76 (-30.75, -28.0238) -> (-20.75, -28.0238)
  line L77 (-20.75, -28.0238) -> (-20.75, -33.0238)
  line L78 (-20.75, -33.0238) -> (20.75, -33.0238)
  line L79 (20.75, -33.0238) -> (20.75, -28.0238)
  line L80 (20.75, -28.0238) -> (30.75, -28.0238)
  line L81 (30.75, -28.0238) -> (41.676, -29.8238)
  line L82 (41.676, -29.8238) -> (44.25, -29.8238)
  line L83 (44.25, -29.8238) -> (44.25, -31.3238)
  line L84 (44.25, -31.3238) -> (41.25, -31.3238)
  line L85 (41.25, -31.3238) -> (30.75, -30.5238)
  line L86 (30.75, -30.5238) -> (23.25, -30.5238)
  line L87 (23.25, -30.5238) -> (23.25, -33.0238)
  line L88 (23.25, -33.0238) -> (28.25, -33.0238)
  line L89 (28.25, -33.0238) -> (28.25, -35.5238)
  line L90 (28.25, -35.5238) -> (53.25, -35.5238) construction
  line L91 (53.25, -35.5238) -> (53.25, -31.3238)
  line L92 (53.25, -31.3238) -> (50.25, -31.3238)
  line L93 (50.25, -31.3238) -> (50.25, -29.8238)
  line L94 (50.25, -29.8238) -> (67.7328, -29.8238)
  arc A11 (67.7328, -29.8238) -> (78, -22.5036) centre (53.25, 1.35) ccw
  line L95 (29.089, 25.8) -> (-29.089, 25.8)
  arc A12 (-29.089, 25.8) -> (-78, 25.2036) centre (-53.25, 1.35) ccw
  line L96 (-67.7328, -29.8238) -> (-50.25, -29.8238)
  line L97 (-50.25, -29.8238) -> (-50.25, -31.3238)
  line L98 (52.75, -35.7238) -> (28.75, -35.7238) construction
  line L99 (52.75, -35.7238) -> (52.75, -36.0238)
  line L100 (51.0833, -35.7238) -> (51.0833, -36.0238)
  line L101 (49.4167, -35.7238) -> (49.4167, -36.0238)
  line L102 (47.75, -35.7238) -> (47.75, -36.0238)
  line L103 (46.0833, -35.7238) -> (46.0833, -36.0238)
  line L104 (44.4167, -35.7238) -> (44.4167, -36.0238)
  line L105 (42.75, -35.7238) -> (42.75, -36.0238)
  line L106 (41.0833, -35.7238) -> (41.0833, -36.0238)
  line L107 (39.4167, -35.7238) -> (39.4167, -36.0238)
  line L108 (37.75, -35.7238) -> (37.75, -36.0238)
  line L109 (36.0833, -35.7238) -> (36.0833, -36.0238)
  line L110 (34.4167, -35.7238) -> (34.4167, -36.0238)
  line L111 (32.75, -35.7238) -> (32.75, -36.0238)
  line L112 (31.0833, -35.7238) -> (31.0833, -36.0238)
  line L113 (29.4167, -35.7238) -> (29.4167, -36.0238)
  line L114 (27.75, -35.7238) -> (27.75, -36.0238)
  line L115 (51.0833, -35.7238) -> (49.4167, -35.7238)
  line L116 (47.75, -35.7238) -> (46.0833, -35.7238)
  line L117 (44.4167, -35.7238) -> (42.75, -35.7238)
  line L118 (41.0833, -35.7238) -> (39.4167, -35.7238)
  line L119 (37.75, -35.7238) -> (36.0833, -35.7238)
  line L120 (34.4167, -35.7238) -> (32.75, -35.7238)
  line L121 (31.0833, -35.7238) -> (29.4167, -35.7238)
  line L122 (-51.0833, -35.7238) -> (-51.0833, -36.0238)
  line L123 (-51.0833, -35.7238) -> (-49.4167, -35.7238)
  line L124 (-49.4167, -35.7238) -> (-49.4167, -36.0238)
  line L125 (-47.75, -35.7238) -> (-47.75, -36.0238)
  line L126 (-47.75, -35.7238) -> (-46.0833, -35.7238)
  line L127 (-46.0833, -35.7238) -> (-46.0833, -36.0238)
  line L128 (-44.4167, -35.7238) -> (-44.4167, -36.0238)
  line L129 (-44.4167, -35.7238) -> (-42.75, -35.7238)
  line L130 (-42.75, -35.7238) -> (-42.75, -36.0238)
  line L131 (-41.0833, -35.7238) -> (-41.0833, -36.0238)
  line L132 (-41.0833, -35.7238) -> (-39.4167, -35.7238)
  line L133 (-39.4167, -35.7238) -> (-39.4167, -36.0238)
  line L134 (-37.75, -35.7238) -> (-37.75, -36.0238)
  line L135 (-37.75, -35.7238) -> (-36.0833, -35.7238)
  line L136 (-36.0833, -35.7238) -> (-36.0833, -36.0238)
  line L137 (-34.4167, -35.7238) -> (-34.4167, -36.0238)
  line L138 (-34.4167, -35.7238) -> (-32.75, -35.7238)
  line L139 (-32.75, -35.7238) -> (-32.75, -36.0238)
  line L140 (-31.0833, -35.7238) -> (-31.0833, -36.0238)
  line L141 (-31.0833, -35.7238) -> (-29.4167, -35.7238)
  line L142 (-29.4167, -35.7238) -> (-29.4167, -36.0238)
  line L143 (78, -22.5036) -> (78, 25.2036)
  arc A13 (78, 25.2036) -> (29.089, 25.8) centre (53.25, 1.35) ccw
  line L144 (-78, 25.2036) -> (-78, -22.5036)
  arc A14 (-78, -22.5036) -> (-67.7328, -29.8238) centre (-53.25, 1.35) ccw
  point P0 (-49.75, -28.0238)
  point P1 (-44.75, -28.0238)
  dimension "d151" = 0.25
  dimension "d153" = 0.25
  dimension "d154" = 0.25
  dimension "d156" = 0.5
  dimension "d157" = 2.5
  dimension "d161" = 1.5
  dimension "d164" = 0.5
  dimension "d165" = 0.6
  dimension "d168" = 0.5
  dimension "d169" = 0.3
  dimension "d172" = -25
  dimension "d173" = 0
  dimension "d237" = 1.5
  constraint perpendicular L11 L12
  constraint perpendicular L12 L13
  constraint perpendicular L11 L14
  constraint perpendicular L14 L15
  constraint perpendicular L10 L16
  constraint perpendicular L16 L21
  constraint perpendicular L21 L22
  constraint perpendicular L20 L23
  constraint perpendicular L15 L24
  constraint collinear L21 L24
  constraint symmetric L1.start L25 L51.end
  constraint symmetric L1.end L25 L0.start
  constraint symmetric L2.start L25 L51.start
  constraint symmetric L3.start L25 L30.end
  constraint symmetric L3.end L25 L27.end
  constraint symmetric L4.start L25 L28.end
  constraint symmetric L5.start L25 L28.start
  constraint symmetric L6.start L25 L31.end
  constraint symmetric L7.start L25 L0.end
  constraint symmetric L7.end L25 L29.end
  constraint symmetric L10.start L25 L35.end
  constraint symmetric L10.end L25 L33.start
  constraint symmetric L11.end L25 L33.end
  constraint symmetric L12.end L25 L34.start
  constraint symmetric L13.end L25 L34.end
  constraint symmetric L14.end L25 L36.end
  constraint symmetric L15.end L25 L32.end
  constraint symmetric L16.start L25 L35.start
  constraint symmetric L17.start L25 L38.start
  constraint symmetric L17.end L25 P1
  constraint symmetric L18.end L25 P0
  constraint symmetric L19.start L25 L49.start
  constraint symmetric L19.end L25 L50.start
  constraint symmetric L20.end L25 L49.end
  constraint symmetric L21.end L25 L37.end
  constraint symmetric L23.end L25 L32.start
  constraint perpendicular L10 L99
  constraint symmetric L25 L100.start L122.start
  constraint symmetric L25 L100.end L122.end
  constraint symmetric L25 L101.start L123.end
  constraint symmetric L25 L101.end L124.end
  constraint symmetric L25 L102.start L125.start
  constraint symmetric L25 L102.end L125.end
  constraint symmetric L25 L103.start L126.end
  constraint symmetric L25 L103.end L127.end
  constraint symmetric L25 L104.start L128.start
  constraint symmetric L25 L104.end L128.end
  constraint symmetric L25 L105.start L129.end
  constraint symmetric L25 L105.end L130.end
  constraint symmetric L25 L106.start L131.start
  constraint symmetric L25 L106.end L131.end
  constraint symmetric L25 L107.start L132.end
  constraint symmetric L25 L107.end L133.end
  constraint symmetric L25 L108.start L134.start
  constraint symmetric L25 L108.end L134.end
  constraint symmetric L25 L109.start L135.end
  constraint symmetric L25 L109.end L136.end
  constraint symmetric L25 L110.start L137.start
  constraint symmetric L25 L110.end L137.end
  constraint symmetric L25 L111.start L138.end
  constraint symmetric L25 L111.end L139.end
  constraint symmetric L25 L112.start L140.start
  constraint symmetric L25 L112.end L140.end
  constraint symmetric L25 L113.start L141.end
  constraint symmetric L25 L113.end L142.end
  measures "d151" distance of L8 L12
  measures "d153" distance of L6 L13
  measures "d154" distance of L5 L14
  measures "d156" distance of L1 L16
  measures "d157" distance of L11 L15
  measures "d161" distance of L10 L24
  measures "d164" distance of L11 L89
  measures "d165" distance of L64 L84
  measures "d168" distance of L9 L10
combine "Kombinieren1" operation add target body 4 tool bodies 8 9 10 11
extrude "Extrusion14" add sketch "Skizze9" along normal blind 7.7 separate body contours L10 L11 L12 L13 L14 L15 L16 L19 L20 L21 L22 L23 L24 L99 L100 L101 L102 L103 L104 L105 L106 L107 L108 L109 L110 L111 L112 L113 L115 L116 L117 L118 L119 L120 L121 | L32 L33 L34 L35 L36 L37 L40 L41 L49 L50 L53 L57 L59 L122 L123 L124 L125 L126 L127 L128 L129 L130 L131 L132 L133 L134 L135 L136 L137 L138 L139 L140 L141 L142 makes body 14 at (-40.25, 34.5238, 17.1333) makes body 15 at (40.25, 34.5238, 17.1333)
extrude "Extrusion15" cut sketch "Skizze8" against normal blind 2.5 contours L2 L11 L12 L13 L14 | L2 L4 L5 L6 L7 bodies 4
extrude "Extrusion16" cut sketch "Skizze8" against normal blind 1.05 contours L2 L6 L19 L20 L21 | L2 L4 L5 L7 L18 L19 L21 bodies 1 2 4
chamfer "Fase1" distance 1.05 distance2 2.2 6 edges at (19, 35.5238, 10) (11.75, 35.5238, 8.5) (4.5, 35.5238, 10) (11.75, 35.5238, 17.5) (19, 35.5238, 14.5) (4.5, 35.5238, 14.5) measured on face at (19, 35.1738, 9.5) measured on face at (9.3333, 35.1738, 8.5) measured on face at (4.5, 35.1738, 10.5) measured on face at (14.1667, 35.1738, 17.5) measured on face at (19, 35.1738, 13.5) measured on face at (4.5, 35.1738, 15.5) tangent chain off on bodies 2 4
extrude "Extrusion20" add sketch "Skizze8" against normal blind 9.5 contours L2 L11 L12 L14 L27 L28 L29 L30 L31 L32 L33 bodies 4
extrude "Extrusion17" add sketch "Skizze4" along normal blind 7 contours A2 | A4 bodies 3
sketch "Skizze10" plane through (0, 0, 17) normal (0, 0, 1) x (-1, 0, 0)
  circle A0 centre (-37.1, -16.85) radius 2.5
  circle A1 centre (-37.1, -16.85) radius 4
  circle A2 centre (-69.7, -16.85) radius 2.5
  circle A3 centre (-69.7, -16.85) radius 4
  circle A4 centre (-37.1, -16.85) radius 2.25
  circle A5 centre (-69.7, -16.85) radius 2.25
  dimension "d210" = 1.5
  dimension "d211" = 1.5
extrude "Extrusion18" add sketch "Skizze10" along normal blind 6.7 separate body contours A4 | A5 makes body 16 at (36.4906, 14.6841, 21.4667) makes body 17 at (67.4612, 17.074, 19.2333)
extrude "Extrusion19" add sketch "Skizze10" along normal blind 2.7 contours A0 | A1 | A2 | A3 bodies 17 16
extrude "Extrusion23" add sketch "Skizze8" against normal blind 11.1 contours L35 L36 A2 L37 bodies 2 1
extrude "Extrusion24" cut sketch "Skizze8" against normal blind 1.5 contours A0 bodies 2
chamfer "Fase3" distance 1.5 distance2 2 1 edges at (-9.1395, 35.5238, 6.9342) measured on face at (-14.5361, 35.0238, 5.6429) on bodies 2
fillet "Abrundung1" radius 2.5 8 edges at (0, -28.3, 0) (87.5532, -14.8764, 0) (0, 35.5238, 0) (-87.5532, -14.8764, 0) (0, -28.3, 22.2) (87.5532, -14.8764, 22.2) (0, 35.5238, 22.2) (-87.5532, -14.8764, 22.2) on bodies 2 4
chamfer "Fase2" distance 0.65 angle 45 1 edges at (-1.3985, 19.9924, 6.25) on bodies 1 2
chamfer "Fase2" distance 0.65 angle 45 1 edges at (68.9346, -17.948, 6.25) on bodies 1 2
chamfer "Fase2" distance 0.65 angle 45 1 edges at (-71.2654, -17.948, 6.25) on bodies 1 2
fillet "Abrundung2" radius 2.5 7 edges at (0, -25.8, 2.5) (66.6965, 30.2846, 2.5) (53.6691, -35.7212, 2.5) (-34.9, 33.0238, 2.5) (23.15, 33.0238, 2.5) (-66.6965, 30.2846, 2.5) (-53.6691, -35.7212, 2.5) on bodies 2
fillet "Abrundung3" radius 2.5 5 edges at (53.6691, -35.7212, 19.7) (73.2049, 26.6385, 19.7) (0, -25.8, 19.7) (-53.6691, -35.7212, 19.7) (-73.2049, 26.6385, 19.7) on bodies 4
fillet "Abrundung3" radius 2.5 2 edges at (7.8, 33.0238, 19.7) (-19.55, 33.0238, 19.7) on bodies 4
extrude "Extrusion25" add sketch "Skizze3" along normal blind 11.6 contours A4 | A6 | A9 bodies 2
extrude "Extrusion26" add sketch "Skizze3" along normal blind 7.5 contours A5 | A7 | A8 bodies 2
extrude "Extrusion27" add sketch "Skizze7" against normal blind 13.1 contours A7 | A9 | A11 bodies 4
combine "Kombinieren2" operation add target body 4 tool bodies 12 13
extrude "Extrusion31" add sketch "Skizze7" against normal blind 6.15 contours L25 L74 L75 L76 bodies 4
extrude "Extrusion32" add sketch "Skizze7" against normal blind 7.7 contours L76 L77 L78 L79 bodies 4
chamfer "Fase4" distance 1 angle 45 2 edges at (-84.6019, -0.5243, 11.5) (81.8981, -0.5243, 11.5) on bodies 4
equation "Board_Width = 150 mm"
equation "Board_Height = 46.6 mm"
equation "Board_MountHoles_Dia = 3.2 mm"
equation "Screw_Dia = 3 mm"
equation "Screw_Head_Dia = 5.5 mm"
equation "Screw_length1 = 7.8 mm" comment "komplett inkl. Kopf"
equation "Screw_Length2 = 16.5 mm" comment "komplett inkl. Kopf"
equation "Button_Dia = 12.5 mm"
equation "d9 = Board_Width / 2"
equation "d10 = Board_Height / 2"
equation "d11 = Board_Width"
equation "d12 = Board_Height"
equation "Button_S_Dia = 5 mm"
equation "d16 = Board_MountHoles_Dia"
equation "d19 = Board_MountHoles_Dia / 2"
equation "d20 = Board_MountHoles_Dia"
equation "d21 = Button_S_Width"
equation "d22 = Button_S_Width"
equation "d25 = Button_S_Dia"
equation "d26 = Button_S_Width"
equation "d27 = Button_S_Width"
equation "d30 = Button_S_Dia"
equation "Button_S_Width = 5.9 mm"
equation "Button_Width = 11.9 mm"
equation "d33 = Button_Width"
equation "d34 = Button_Width"
equation "d37 = Button_Width"
equation "d38 = Button_Width"
equation "d39 = Button_Width"
equation "d40 = Button_Width"
equation "d41 = Button_Width"
equation "d42 = Button_Width"
equation "d47 = Button_Dia"
equation "d48 = Button_Dia"
equation "d49 = Button_Dia"
equation "d50 = Button_Dia"
equation "Joystick_Dia = 30 mm"
equation "d56 = Joystick_Dia"
equation "Wall_Thickness = 2.5 mm"
equation "d59 = Wall_Thickness + 1.5 mm"
equation "d60 = Wall_Thickness + 2.5 mm"
equation "d61 = -Wall_Thickness"
equation "d62 = Screw_Dia - 0.5 mm"
equation "d63 = Screw_Head_Dia + 0.5 mm"
equation "d64 = Screw_Dia"
equation "d65 = Screw_Head_Dia + 0.5 mm"
equation "d66 = Screw_Head_Dia + 0.5 mm"
equation "d67 = Screw_Dia - 0.5 mm"
equation "Screw_Standoff_Height_Below = 5 mm"
equation "d69 = Wall_Thickness"
equation "d70 = Wall_Thickness"
equation "d71 = Wall_Thickness"
equation "d72 = Wall_Thickness"
equation "d74 = 2 * Wall_Thickness + Screw_Standoff_Height_Below"
equation "d76 = Screw_Standoff_Height_Below + Wall_Thickness / 2"
equation "Ctrl_Height = Board_Thickness + 2 * Wall_Thickness + Screw_Standoff_Height_Below"
equation "Board_Thickness = 12.2 mm" comment "inkl.Platz für Taster"
equation "d80 = USB_Port_Height"
equation "d82 = Board_PCB_Thickness"
equation "d87 = 1.8 mm"
equation "Board_PCB_Thickness = 1.6 mm"
equation "USB_Port_Height = Wall_Thickness + Screw_Standoff_Height_Below + Board_PCB_Thickness + 0.2 mm + Micro_Thickness_aber_nicht_der_echte" comment "höhe des ports am controller"
equation "Micro_Thickness_aber_nicht_der_echte = 4 mm - d87" comment "?"
equation "d106 = Ctrl_Height"
equation "d107 = Screw_Dia"
equation "d109 = Screw_Dia"
equation "d110 = Screw_Dia + Wall_Thickness * 2"